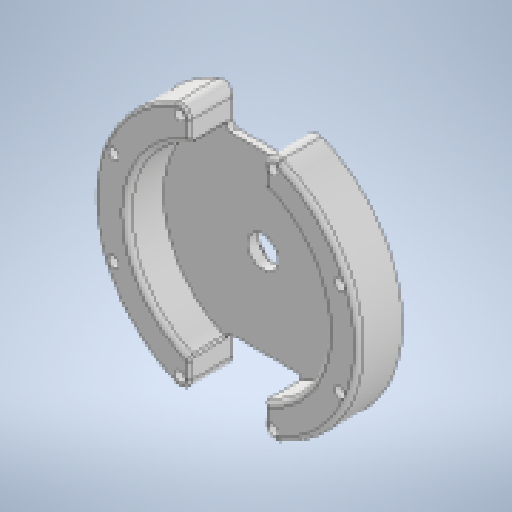
# Autodesk Inventor part: basefixpart_forR3
Saved by Autodesk Inventor 2024 (Build 280153000, 153)
## iProperties
Created: 2025-05-24
Part Number: basefixpart_forR3
Material: 一般
Document SubType Name: Modeling
Designer: kshau
Density: 1 g/cm^3
Appearance: 既定
Mass: 77.9972 g
Surface Area: 271.132 cm^2
Volume: 77.9972 cm^3
Author: kshau
Autodesk Inventor part; units mm, degrees
ref_plane "YZ Plane" through (0, 0, 0) normal (1, 0, 0) x (0, 1, 0)
ref_plane "XZ Plane" through (0, 0, 0) normal (0, 1, 0) x (-1, 0, 0)
ref_plane "XY Plane" through (0, 0, 0) normal (0, 0, 1) x (1, 0, 0)
sketch "スケッチ1" plane through (0, 0, 0) normal (0, 0, 1) x (1, 0, 0)
  circle A0 centre (0, 0) radius 53
  line L0 (0, 0) -> (53, 0)
  line L1 (0, 0) -> (39.7995, 35)
  line L2 (39.7995, 35) -> (0, 35)
  line L3 (0, 0) -> (0, 53)
  line L4 (-39.7995, 35) -> (0, 35)
  line L5 (39.7995, -35) -> (0, -35)
  line L6 (-39.7995, -35) -> (0, -35)
  line L7 (15, -35) -> (15, -50.8331)
  line L8 (-15, -35) -> (-15, -50.8331)
  line L9 (15, 35) -> (15, 50.8331)
  line L10 (-15, 35) -> (-15, 50.8331)
  point P0 (-39.7995, 35)
  point P1 (-39.7995, -35)
  point P2 (39.7995, -35)
  dimension "d0" = 106
  dimension "d20" = 15
  dimension "d21" = 35
  constraints: 22 end point, 10 symmetric about line, 4 point on circle, 2 horizontal, 1 centre point, 1 coincident, 1 perpendicular, 1 point on line, 1 vertical
  measures "d0" diameter of A0
  measures "d20" distance between parallel lines of L3 L7
  measures "d21" distance between parallel lines of L0 L2
extrude "押し出し1" add sketch "スケッチ1" along normal blind 19.5 contours L0 L1 A0 | A0 L5 L6 L4 L3 L0 | L2 L9 A0 | L1 L3 L2 | A0 L7 L5 | A0 L6 L8 | L4 A0 L10
sketch "スケッチ2" plane through (0, 0, 19.5) normal (0, 0, 1) x (1, 0, 0)
  circle A0 centre (0, 0) radius 39.95
  dimension "d4" = 79.9
  constraints: 1 centre point, 1 coincident
  measures "d4" diameter of A0
extrude "押し出し2" cut sketch "スケッチ2" against normal blind 14.6
sketch "スケッチ3" plane through (0, 0, 0) normal (0, 0, -1) x (-1, 0, 0)
  circle A0 centre (0, 0) radius 49
  line L0 (0, 0) -> (-49, 0)
  line L1 (0, 0) -> (-45.2701, -18.7515)
  point P0 (-18.7515, -45.2701)
  point P1 (18.7515, -45.2701)
  point P2 (45.2701, -18.7515)
  point P3 (45.2701, 18.7515)
  point P4 (18.7515, 45.2701)
  point P5 (-18.7515, 45.2701)
  point P6 (-45.2701, 18.7515)
  dimension "d7" = 98
  dimension "d8" = 22.5
  dimension "d11" = 360
  constraints: 4 end point, 2 coincident, 2 point on circle, 1 centre point, 1 horizontal, 9 other
  measures "d7" diameter of A0
  measures "d8" angle of L0 L1
hole "穴1" at (45.2701, -18.7515, 0) at (18.7515, -45.2701, 0) at (-18.7515, -45.2701, 0) at (-45.2701, -18.7515, 0) at (-45.2701, 18.7515, 0) at (-18.7515, 45.2701, 0) at (18.7515, 45.2701, 0) at (45.2701, 18.7515, 0) direction (0, 0, 1) diameter 4.2 end through all
fillet "フィレット1" radius 4 4 edges at (-15, 50.8331, 9.75) (15, 50.8331, 9.75) (15, -50.8331, 9.75) (-15, -50.8331, 9.75)
fillet "フィレット2" radius 2 4 edges at (-15, 35, 2.45) (15, 35, 2.45) (15, -35, 2.45) (-15, -35, 2.45)
sketch "スケッチ4" plane through (0, 0, 0) normal (0, 0, -1) x (-1, 0, 0)
  arc A0 (-15, 37.0271) -> (-15, -37.0271) centre (0, 0) ccw projected
  circle A1 centre (0, 0) radius 23.5
  point P0 (14.9998, 36.9732)
  point P1 (14.9998, -36.9732)
  dimension "d24" = 47
  constraints: 1 centre point, 1 coincident
  measures "d24" diameter of A1
extrude "押し出し3" add sketch "スケッチ4" along normal blind 4
sketch "スケッチ5" plane through (0, 0, -4) normal (0, 0, -1) x (-1, 0, 0)
  point P0 (0, 0)
  point P1 (0, 0)
  constraints: 1 coincident
hole "穴2" at (0, 0, -4) direction (0, 0, 1) diameter 12.2 end through all
sketch "スケッチ6" plane through (0, 0, -4) normal (0, 0, -1) x (-1, 0, 0)
  circle A0 centre (0, 0) radius 6.1 projected
  circle A1 centre (0, 0) radius 11.1
  dimension "d34" = 22.2
  constraints: 1 centre point, 1 coincident
  measures "d34" diameter of A1
extrude "押し出し4" cut sketch "スケッチ6" against normal blind 4.8
sketch "スケッチ7" plane through (0, 0, 0) normal (0, 0, -1) x (-1, 0, 0)
  circle A0 centre (0, 0) radius 53
  circle A1 centre (0, 0) radius 6.1 projected
  circle A2 centre (0, 0) radius 32.75
  dimension "d37" = 106
  dimension "d38" = 65.5
  constraints: 2 centre point, 2 coincident
  measures "d37" diameter of A0
  measures "d38" diameter of A2
extrude "押し出し5" cut sketch "スケッチ7" against normal blind 2 contours A0
fillet "フィレット3" radius 2 2 edges at (23.5, 0, 0) (32.75, 0, 2)
fillet "フィレット4" radius 2 7 edges at (16.7869, 48.4983, 19.5) (15, 41.0967, 19.5) (16.7869, -48.4983, 19.5) (15, -41.0967, 19.5) (53, 0, 19.5) (39.95, 0, 19.5) (-39.95, 0, 19.5)
fillet "フィレット5" radius 1 9 edges at (-15, -37.0271, 11.2) (-15, -42.1715, 19.5) (-16.7869, -48.4983, 19.5) (-53, 0, 19.5) (-16.7869, 48.4983, 19.5) (-15, 42.1715, 19.5) (-15, 37.68, 18.9341) (-15, 37.0271, 11.2) (-15, -37.68, 18.9341)
fillet "フィレット7" radius 1 1 edges at (11.1, 0, -4)
